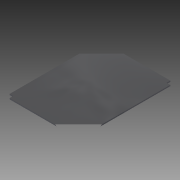
# Autodesk Inventor part: ElectronicsEnclosureBottom
Saved by Autodesk Inventor 2015 (Build 190159000, 159)
## iProperties
Created: 2014-10-21
Part Number: ElectronicsEnclosureBottom
Material: ABS Plastic
Document SubType Name: Modeling
Designer: Jack
Density: 1.06 g/cm^3
Appearance: Smooth - Medium Gray
Author: Jack
Autodesk Inventor part; units mm, degrees
ref_plane "YZ Plane" through (0, 0, 0) normal (1, 0, 0) x (0, 1, 0)
ref_plane "XZ Plane" through (0, 0, 0) normal (0, 1, 0) x (-1, 0, 0)
ref_plane "XY Plane" through (0, 0, 0) normal (0, 0, 1) x (1, 0, 0)
sketch "Sketch1" plane through (0, 0, 0) normal (0, 0, 1) x (1, 0, 0)
  line L0 (19, -40) -> (19, -480) projected
  line L1 (-356, -20) -> (-1, -20) projected
  line L2 (-376, -40) -> (-376, -480) projected
  line L3 (-356, -500) -> (-1, -500) projected
  line L4 (19, -40) -> (19, -20)
  line L5 (19, -20) -> (-1, -20)
  line L6 (-356, -20) -> (-376, -20)
  line L7 (-376, -20) -> (-376, -40)
  line L8 (-376, -480) -> (-376, -500)
  line L9 (-376, -500) -> (-356, -500)
  line L10 (-1, -500) -> (19, -500)
  line L11 (19, -480) -> (19, -500)
  point P0 (0, 0)
  constraints: 16 end point, 4 perpendicular, 4 point on line, 1 vertical
extrude "Extrusion1" add sketch "Sketch1" along normal blind 6
sketch "Sketch3" plane through (0, 0, 6) normal (0, 0, 1) x (1, 0, 0)
  line L0 (19, -500) -> (19, -20) projected
  line L1 (19, -20) -> (-376, -20) projected
  line L2 (-376, -20) -> (-376, -500) projected
  line L3 (-376, -500) -> (19, -500) projected
  line L4 (-369.3, -40) -> (-375, -40) projected
  line L5 (-356, -21) -> (-356, -26.7) projected
  line L6 (-1, -21) -> (-1, -26.7) projected
  line L7 (12.3, -40) -> (18, -40) projected
  line L8 (12.3, -480) -> (18, -480) projected
  line L9 (-1, -499) -> (-1, -493.3) projected
  line L10 (-356, -493.3) -> (-356, -499) projected
  line L11 (-369.3, -480) -> (-375, -480) projected
  line L12 (-376, -480) -> (-356, -480)
  line L13 (-356, -480) -> (-356, -500)
  line L14 (-1, -500) -> (-1, -480)
  line L15 (-1, -480) -> (19, -480)
  line L16 (-1, -20) -> (-1, -40)
  line L17 (-1, -40) -> (19, -40)
  line L18 (-356, -20) -> (-356, -40)
  line L19 (-356, -40) -> (-376, -40)
  point P0 (0, 0)
  point P1 (-356, -23.85)
  constraints: 20 point on line, 16 end point, 3 perpendicular, 2 vertical, 1 midpoint
extrude "Extrusion2" cut sketch "Sketch3" against normal up to next contours L3 L14 L9 L15 L8 L0 | L15 L8 L14 L9 L3 L13 L10 L12 L11 L2 L19 L4 L18 L5 L1 L16 L6 L17 L7 L0 | L3 L2 L12 L11 L13 L10 | L18 L5 L19 L4 L2 L1
body "Solid1"
